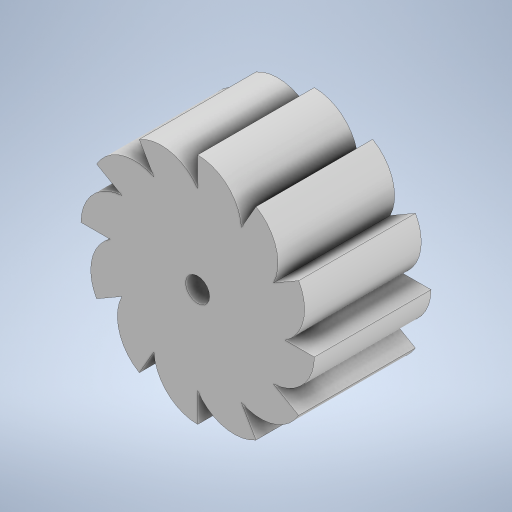
# Autodesk Inventor part: THE_WHEEL 2.0
Saved by Autodesk Inventor 2023 (Build 270158000, 158)
## iProperties
Created: 2023-01-26
Part Number: THE_WHEEL 2.0
Material: Generic
Document SubType Name: Modeling
Designer: Steven
Density: 1 g/cm^3
Appearance: Default
Author: Steven
Autodesk Inventor part; units mm, degrees
ref_plane "YZ Plane" through (0, 0, 0) normal (1, 0, 0) x (0, 1, 0)
ref_plane "XZ Plane" through (0, 0, 0) normal (0, 1, 0) x (-1, 0, 0)
ref_plane "XY Plane" through (0, 0, 0) normal (0, 0, 1) x (1, 0, 0)
sketch "Sketch1" plane through (0, 0, 0) normal (0, 0, 1) x (1, 0, 0)
  circle A0 centre (0, 0) radius 25.4 construction
  circle A1 centre (0, 0) radius 19.05
  arc A2 (19.05, 0) -> (21.997, 12.7) centre (13.7293, 7.9266) ccw
  circle A3 centre (0, 0) radius 2.6035
  line L0 (0, 0) -> (19.05, 0) construction
  line L1 (0, 0) -> (21.997, 12.7) construction
  line L2 (21.997, 12.7) -> (16.4978, 9.525)
  line L3 (12.7, 21.997) -> (9.525, 16.4978)
  arc A4 (16.4978, 9.525) -> (12.7, 21.997) centre (7.9266, 13.7293) ccw
  line L4 (0, 25.4) -> (0, 19.05)
  arc A5 (9.525, 16.4978) -> (0, 25.4) centre (0, 15.8532) ccw
  line L5 (-12.7, 21.997) -> (-9.525, 16.4978)
  arc A6 (0, 19.05) -> (-12.7, 21.997) centre (-7.9266, 13.7293) ccw
  line L6 (-21.997, 12.7) -> (-16.4978, 9.525)
  arc A7 (-9.525, 16.4978) -> (-21.997, 12.7) centre (-13.7293, 7.9266) ccw
  line L7 (-25.4, 0) -> (-19.05, 0)
  arc A8 (-16.4978, 9.525) -> (-25.4, 0) centre (-15.8532, 0) ccw
  line L8 (-21.997, -12.7) -> (-16.4978, -9.525)
  arc A9 (-19.05, 0) -> (-21.997, -12.7) centre (-13.7293, -7.9266) ccw
  line L9 (-12.7, -21.997) -> (-9.525, -16.4978)
  arc A10 (-16.4978, -9.525) -> (-12.7, -21.997) centre (-7.9266, -13.7293) ccw
  line L10 (0, -25.4) -> (0, -19.05)
  arc A11 (-9.525, -16.4978) -> (0, -25.4) centre (0, -15.8532) ccw
  line L11 (12.7, -21.997) -> (9.525, -16.4978)
  arc A12 (0, -19.05) -> (12.7, -21.997) centre (7.9266, -13.7293) ccw
  line L12 (21.997, -12.7) -> (16.4978, -9.525)
  arc A13 (9.525, -16.4978) -> (21.997, -12.7) centre (13.7293, -7.9266) ccw
  line L13 (25.4, 0) -> (19.05, 0)
  arc A14 (16.4978, -9.525) -> (25.4, 0) centre (15.8532, 0) ccw
  point P0 (9.525, 16.4978)
  point P1 (0, 19.05)
  point P2 (-9.525, 16.4978)
  point P3 (-16.4978, 9.525)
  point P4 (-19.05, 0)
  point P5 (-16.4978, -9.525)
  point P6 (-9.525, -16.4978)
  point P7 (0, -19.05)
  point P8 (9.525, -16.4978)
  point P9 (16.4978, -9.525)
  point P10 (19.05, 0)
  point P11 (16.4978, 9.525)
  dimension "d0" = 50.8
  dimension "d1" = 38.1
  dimension "d11" = 5.207
  dimension "d17" = 30
  dimension "d20" = 360
  constraints: 28 end point, 26 point on circle, 14 centre point, 3 coincident, 1 horizontal, 1 point on line, 77 other
  measures "d1" diameter of A1
  measures "d11" diameter of A3
  measures "d17" angle of L1 L0
extrude "Extrusion1" add sketch "Sketch1" along normal blind 25.4
body "Solid1"
